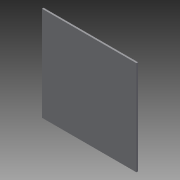
# Autodesk Inventor part: Platte6mm
Saved by Autodesk Inventor 2015 (Build 190159000, 159)
## iProperties
Created: 2016-04-07
Part Number: Platte6mm
Material: Generisch
Document SubType Name: Modeling
Designer: Carl
Density: 1 g/cm^3
Appearance: Vorgabe
Author: Carl
Autodesk Inventor part; units mm, degrees
ref_plane "YZ Plane" through (0, 0, 0) normal (1, 0, 0) x (0, 1, 0)
ref_plane "XZ Plane" through (0, 0, 0) normal (0, 1, 0) x (-1, 0, 0)
ref_plane "XY Plane" through (0, 0, 0) normal (0, 0, 1) x (1, 0, 0)
sketch "Skizze1" plane through (0, 0, 0) normal (0, 1, 0) x (-1, 0, 0)
  line L0 (176, -176) -> (-176, -176)
  line L1 (-176, -176) -> (-176, 176)
  line L2 (-176, 176) -> (176, 176)
  line L3 (176, 176) -> (176, -176)
  line L4 (176, -176) -> (-176, 176) construction
  line L5 (-176, -176) -> (176, 176) construction
  point P0 (0, 0)
  dimension "d0" = 352
  dimension "d1" = 352
  constraints: 12 end point, 2 midpoint, 2 parallel, 1 horizontal, 1 perpendicular
  measures "d0" distance of L1.end L2.end
  measures "d1" distance of L0.end L1.end
extrude "Extrusion1" add sketch "Skizze1" along normal blind 6
equation "\"d1\" = d0"
